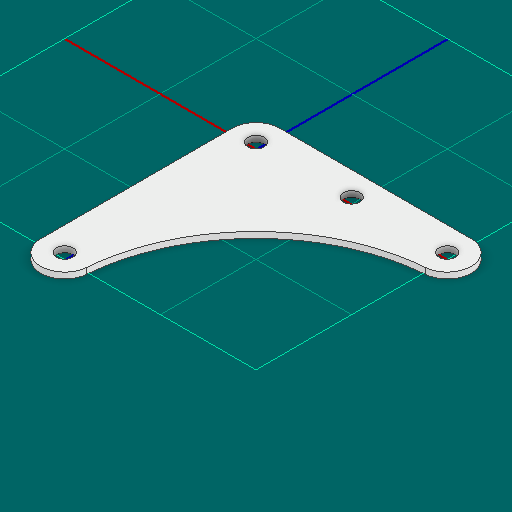
# Autodesk Inventor part: Arm Triangle Gusset
Saved by Autodesk Inventor 2025 (Build 290162000, 162)
## iProperties
Created: 2024-10-21
Part Number: Arm Triangle Gusset
Material: Acetal Resin, White
Document SubType Name: Modeling
Designer: averey
Density: 1.425 g/cm^3
Appearance: Smooth - White
Author: averey
Autodesk Inventor part; units mm, degrees
ref_plane "YZ Plane" through (0, 0, 0) normal (1, 0, 0) x (0, 1, 0)
ref_plane "XZ Plane" through (0, 0, 0) normal (0, 1, 0) x (-1, 0, 0)
ref_plane "XY Plane" through (0, 0, 0) normal (0, 0, 1) x (1, 0, 0)
sketch "main" plane through (0, 0, 0) normal (0, 0, 1) x (1, 0, 0)
  circle A0 centre (27.8145, 23.5161) radius 2.1844
  circle A1 centre (27.8145, -27.2839) radius 2.1844
  circle A2 centre (-22.9855, -27.2839) radius 2.1844
  arc A3 (-23.5053, -20.9552) -> (-22.9855, -33.6339) centre (-22.9855, -27.2839) ccw
  arc A4 (27.8145, -33.6339) -> (34.1645, -27.2839) centre (27.8145, -27.2839) ccw
  arc A5 (34.1645, 23.5161) -> (21.4858, 24.0358) centre (27.8145, 23.5161) ccw
  line L0 (34.1645, 23.5161) -> (34.1645, -27.2839)
  line L1 (27.8145, -33.6339) -> (-22.9855, -33.6339)
  arc A6 (-23.5053, -20.9552) -> (21.4858, 24.0358) centre (-27.5308, 28.0614) ccw
  point P0 (11.2944, -10.7639)
sketch "Sketch1" plane through (0, 0, 0) normal (0, 1, 0) x (-1, 0, 0)
  circle A0 centre (-25.4, 0) radius 2.1844
  circle A1 centre (0, 50.8) radius 2.1844
  circle A2 centre (0, 0) radius 2.1844
  circle A3 centre (-50.8, 0) radius 2.1844
  arc A4 (-51.3197, 6.3287) -> (-50.8, -6.35) centre (-50.8, 0) ccw
  arc A5 (0, -6.35) -> (6.35, 0) centre (0, 0) ccw
  arc A6 (6.35, 50.8) -> (-6.3287, 51.3197) centre (0, 50.8) ccw
  line L0 (6.35, 50.8) -> (6.35, 0)
  line L1 (0, -6.35) -> (-50.8, -6.35)
  arc A7 (-51.3197, 6.3287) -> (-6.3287, 51.3197) centre (-55.3453, 55.3453) ccw
  dimension "d2" = 4.3688
  constraints: 1 centre point, 1 other
  measures "d2" diameter of A0
extrude "Extrusion1" add sketch "Sketch1" along normal blind 1.5875
body "Solid1"
